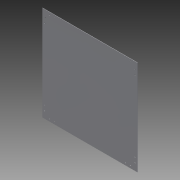
# Autodesk Inventor part: Back Funnel Piece
Saved by Autodesk Inventor 2014 (Build 180170000, 170)
## iProperties
Created: 2014-01-06
Part Number: Back Funnel Piece
Material: Aluminum 6061
Document SubType Name: Modeling
Designer: Michael
Density: 2.71 g/cm^3
Appearance: Aluminum - Flat
Author: Michael
Autodesk Inventor part; units mm, degrees
ref_plane "YZ Plane" through (0, 0, 0) normal (1, 0, 0) x (0, 1, 0)
ref_plane "XZ Plane" through (0, 0, 0) normal (0, 1, 0) x (-1, 0, 0)
ref_plane "XY Plane" through (0, 0, 0) normal (0, 0, 1) x (1, 0, 0)
sketch "Sketch1" plane through (0, 0, 0) normal (0, 0, 1) x (1, 0, 0)
  line L0 (0, 0) -> (508, 0)
  line L1 (508, 0) -> (508, 508)
  line L2 (508, 508) -> (0, 508)
  line L3 (0, 508) -> (0, 0)
  line L4 (0, 254) -> (508, 254) construction
  line L5 (254, 508) -> (254, 0) construction
  circle A0 centre (12.7, 469.9) radius 2.4892
  circle A1 centre (12.7, 444.5) radius 2.4892
  circle A2 centre (12.7, 38.1) radius 2.4892
  circle A3 centre (12.7, 63.5) radius 2.4892
  circle A4 centre (38.1, 12.7) radius 2.4892
  circle A5 centre (63.5, 12.7) radius 2.4892
  circle A6 centre (444.5, 12.7) radius 2.4892
  circle A7 centre (469.9, 12.7) radius 2.4892
  circle A8 centre (495.3, 38.1) radius 2.4892
  circle A9 centre (495.3, 63.5) radius 2.4892
  circle A10 centre (495.3, 444.5) radius 2.4892
  circle A11 centre (495.3, 469.9) radius 2.4892
  circle A12 centre (469.9, 495.3) radius 2.4892
  circle A13 centre (444.5, 495.3) radius 2.4892
  circle A14 centre (63.5, 495.3) radius 2.4892
  circle A15 centre (38.1, 495.3) radius 2.4892
  point P0 (254, 254)
  dimension "d0" = 508
  dimension "d1" = 508
  dimension "d2" = 4.9784
  dimension "d3" = 12.7
  dimension "d4" = 38.1
  dimension "d7" = 25.4
  dimension "d14" = 360
  constraints: 16 centre point, 12 end point, 5 midpoint, 2 parallel, 2 symmetric about line, 1 horizontal, 1 perpendicular, 1 vertical, 37 other
  measures "d0" distance of L2.end L1.end
  measures "d1" distance of L1.end L0.end
  measures "d2" diameter of A0
  measures "d3" distance from line of L3 A0.centre
  measures "d4" distance from line of L2 A0.centre
  measures "d7" distance of A0.centre A1.centre
extrude "Extrusion1" add sketch "Sketch1" along normal blind 1.5875
body "Solid1"
